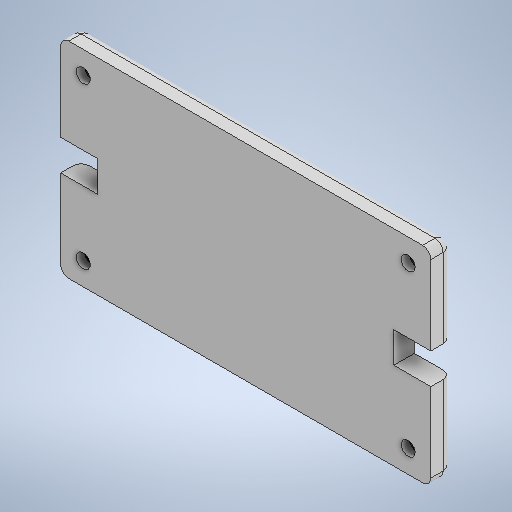
# Autodesk Inventor part: tcs3200_gate_lid
Saved by Autodesk Inventor 2025 (Build 290162000, 162)
## iProperties
Created: 2025-02-06
Part Number: tcs3200_gate_lid
Material: Všeobecné
Document SubType Name: Modeling
Designer: lukas
Density: 1 g/cm^3
Appearance: Výchozí
Author: lukas
## iProperties of the stored document tcs3200_gate_lid_3D tisk.ipt
Created: 2025-02-17
Part Number: tcs3200_gate_lid_3D tisk
Material: Všeobecné
Document SubType Name: Modeling
Designer: lukas
Density: 1 g/cm^3
Appearance: Výchozí
Author: lukas
Autodesk Inventor part; units mm, degrees
ref_plane "YZ Plane" through (0, 0, 0) normal (1, 0, 0) x (0, 1, 0)
ref_plane "XZ Plane" through (0, 0, 0) normal (0, 1, 0) x (-1, 0, 0)
ref_plane "XY Plane" through (0, 0, 0) normal (0, 0, 1) x (1, 0, 0)
sketch "Náčrt1" plane through (0, 0, 0) normal (0, 0, 1) x (1, 0, 0)
  line L0 (0, 35) -> (0, -35) projected
  line L1 (-63, 0) -> (63, 0) projected
  line L2 (-45, 25) -> (45, 25)
  line L3 (45, 25) -> (45, -25)
  line L4 (45, -25) -> (-45, -25)
  line L5 (-45, -25) -> (-45, 25)
  point P0 (0, 0)
  dimension "d0" = 90
  dimension "d1" = 50
  constraints: 8 end point, 2 parallel, 1 horizontal, 1 perpendicular, 2 other
  measures "d0" distance of L2.start L2.end
  measures "d1" distance of L2.end L3.end
extrude "Vysunutí1" add sketch "Náčrt1" along normal blind 5
sketch "Náčrt4" plane through (0, 0, 0) normal (0, 0, -1) x (-1, 0, 0)
  line L0 (45, 25) -> (45, -25) projected
  line L1 (-45, 25) -> (45, 25) projected
  line L2 (-45, -25) -> (-45, 25) projected
  line L3 (45, -25) -> (-45, -25) projected
  line L4 (0, -35) -> (0, 35) projected
  line L5 (-63, 0) -> (63, 0) projected
  point P0 (0, 0)
  point P1 (-39.5, 19.5)
  dimension "d13" = 5.5
  dimension "d14" = 5.5
  measures "d13" distance from line of L2 point (-39.5, 19.5)
  measures "d14" distance from line of L1 point (-39.5, 19.5)
hole "Díra1" at (39.5, 19.5, 0) direction (0, 0, 1) diameter 3.4 end through all counterbore diameter 6.1 counterbore depth 3 clearance for "Strojní šroub se zápustnou hlavou" size "M3" standard "Ansi M metrický profil"
mirror "Zrcadlit2" about plane through (0, 0, 0) normal (0, 1, 0) of "Díra1"
mirror "Zrcadlit3" about plane through (0, 0, 0) normal (1, 0, 0) of "Díra1", "Zrcadlit2"
fillet "Zaoblení2" radius 2 8 edges at (0, 25, 0) (45, 0, 0) (45, 25, 2.5) (0, -25, 0) (45, -25, 2.5) (-45, 0, 0) (-45, -25, 2.5) (-45, 25, 2.5)
sketch "Náčrt6" plane through (0, 0, 0) normal (0, 0, -1) x (-1, 0, 0)
  circle A0 centre (-39.5, 19.5) radius 3.05 projected
  circle A1 centre (-39.5, -19.5) radius 3.05 projected
  circle A2 centre (39.5, 19.5) radius 3.05 projected
  circle A3 centre (39.5, -19.5) radius 3.05 projected
  line L0 (43, -23) -> (-43, -23) projected
  line L1 (43, 23) -> (43, -23) projected
  line L2 (-43, 23) -> (43, 23) projected
  line L3 (-43, -23) -> (-43, 23) projected
  line L4 (-43, 23) -> (-45, 23) projected
  line L5 (-45, 23) -> (-45, -23) projected
  line L6 (-45, -23) -> (-43, -23) projected
  line L7 (-43, -23) -> (-43, 23) projected
  line L8 (-45, 3.75) -> (-36, 3.75)
  line L9 (-36, 3.75) -> (-36, -3.75)
  line L10 (-36, -3.75) -> (-45, -3.75)
  line L11 (-45, -3.75) -> (-45, 3.75)
  line L12 (-63, 0) -> (63, 0) projected
  point P0 (0, 0)
  dimension "d23" = 9
  dimension "d24" = 7.5
  constraints: 8 end point, 2 parallel, 1 horizontal, 1 perpendicular, 1 point on line, 1 other
  measures "d23" distance of L8.start L8.end
  measures "d24" distance between parallel lines of L8 L10
extrude "Vysunutí4" cut sketch "Náčrt6" against normal through all contours L10 L5 L12 L3 | L3 L12 L9 L10 | L12 L3 L8 L9 | L12 L5 L8 L3
mirror "Zrcadlit4" about plane through (0, 0, 0) normal (1, 0, 0) of "Vysunutí4"
